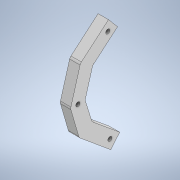
# Autodesk Inventor part: bogie2
Saved by Autodesk Inventor 2020 (Build 240168000, 168)
## iProperties
Created: 2020-05-20
Part Number: bogie2
Material: Generic
Document SubType Name: Modeling
Designer: Manish
Density: 1 g/cm^3
Appearance: Default
Author: Manish
Autodesk Inventor part; units mm, degrees
ref_plane "YZ Plane" through (0, 0, 0) normal (1, 0, 0) x (0, 1, 0)
ref_plane "XZ Plane" through (0, 0, 0) normal (0, 1, 0) x (-1, 0, 0)
ref_plane "XY Plane" through (0, 0, 0) normal (0, 0, 1) x (1, 0, 0)
sketch "Sketch2" plane through (0, 0, 0) normal (1, 0, 0) x (0, 1, 0)
  circle A0 centre (0, 0) radius 3
  line L0 (0, 0) -> (-42.9956, -13.2808)
  line L1 (-42.9956, -13.2808) -> (-74.8971, -51.7814)
  line L2 (0, 0) -> (43.2274, -12.5056)
  line L3 (43.2274, -12.5056) -> (75.6325, -50.5833)
  line L4 (0, 0) -> (-2.961, 9.5861)
  line L5 (0, 0) -> (2.9513, -9.5546)
  line L6 (-42.9956, -13.2808) -> (-46.1884, -2.9442)
  line L7 (-42.9956, -13.2808) -> (-40.0443, -22.8354)
  line L8 (-1.7282, 9.9435) -> (-40.7027, -1.3541)
  line L9 (-30.0445, -19.7466) -> (-1.6206, -10.9668)
  line L10 (-42.9956, -13.2808) -> (-32.8938, -21.6512)
  line L11 (-42.9956, -13.2808) -> (-50.6957, -6.9005)
  line L12 (-32.8938, -21.6512) -> (-64.7954, -60.1517)
  line L13 (-64.7954, -60.1517) -> (-80.1956, -47.3911)
  line L14 (-80.1956, -47.3911) -> (-43.6523, -3.2887)
  line L15 (0, 0) -> (2.779, 9.6061)
  line L16 (0, 0) -> (-2.779, -9.6061)
  line L17 (43.2274, -12.5056) -> (46.0064, -2.8996)
  line L18 (46.0064, -2.8996) -> (40.4484, -22.1117)
  line L19 (1.8176, -10.9359) -> (35.8276, -20.7749)
  line L20 (47.1616, -3.2338) -> (1.6097, 9.9444)
  line L21 (43.2274, -12.5056) -> (50.8429, -6.0246)
  line L22 (43.2274, -12.5056) -> (35.6119, -18.9867)
  line L23 (75.6325, -50.5833) -> (83.2481, -44.1023)
  line L24 (83.2481, -44.1023) -> (68.017, -57.0643)
  line L25 (68.017, -57.0643) -> (38.7295, -22.65)
  line L26 (83.2481, -44.1023) -> (50.0635, -5.1088)
  arc A1 (-40.7027, -1.3541) -> (-43.6523, -3.2887) centre (-39.0322, -7.1169) ccw
  arc A2 (-30.0445, -19.7466) -> (-32.8938, -21.6512) centre (-28.2737, -25.4793) ccw
  arc A3 (1.6097, 9.9444) -> (-1.7282, 9.9435) centre (-0.0577, 4.1807) ccw
  arc A4 (1.8176, -10.9359) -> (-1.6206, -10.9668) centre (0.1501, -16.6995) ccw
  arc A5 (50.0635, -5.1088) -> (47.1616, -3.2338) centre (45.4942, -8.9974) ccw
  arc A6 (38.7295, -22.65) -> (35.8276, -20.7749) centre (34.1601, -26.5386) ccw
  point P0 (2.6602, -14.5039)
  point P1 (16.281, 0.1411)
  point P2 (-48.294, -8.8905)
  dimension "d37" = 6
  dimension "d38" = 45
  dimension "d39" = 10
  dimension "d40" = 20
  dimension "d41" = 50
  dimension "d42" = 10
  dimension "d43" = 10
  dimension "d44" = 10
  dimension "d45" = 20
  dimension "d46" = 10
  dimension "d47" = 10
  dimension "d48" = 10
  dimension "d49" = 20
  dimension "d50" = 6
  dimension "d51" = 6
  dimension "d52" = 50
  dimension "d53" = 10
  dimension "d54" = 1
  dimension "d55" = 33.466
  dimension "d56" = 66.767
  dimension "d57" = 99.956
  dimension "d58" = 75.5671
  dimension "d59" = 77.0952
  dimension "d60" = 22.3248
  dimension "d61" = 74.7699
  dimension "d62" = 42.1891
  constraints: 54 end point, 15 point on line, 14 perpendicular, 12 point on circle, 12 tangent, 7 centre point, 4 equal radius, 3 equal length, 1 coincident
  measures "d37" diameter of A0
  measures "d38" distance between parallel lines of L5 L7
  measures "d39" distance of L0.end L11.end
  measures "d40" distance of L13.start L13.end
  measures "d41" distance between parallel lines of L11 L13
  measures "d42" distance of L16.start L15.end
  measures "d43" distance of L16.start L16.end
  measures "d44" distance of L17.start L17.end
  measures "d45" distance of L17.end L18.end
  measures "d46" distance of L17.start L21.end
  measures "d47" distance of L17.start L22.end
  measures "d48" distance of L3.end L24.start
  measures "d49" distance of L24.start L25.start
  measures "d50" radius of A1
  measures "d51" radius of A3
  measures "d52" distance between parallel lines of L24 L22
  measures "d53" distance between parallel lines of L9 L0
  measures "d54" angle of L0 L8
  measures "d55" angle of L17 L24
  measures "d56" angle of L5 L23
  measures "d57" angle of L10 L23
  measures "d58" distance from line of L24.start L8
  measures "d59" distance from line of point (16.281, 0.141) L24
  measures "d60" distance from line of point (16.281, 0.141) L26
  measures "d61" distance from line of point (2.66, -14.504) L24
  measures "d62" distance from line of point (2.66, -14.504) L26
extrude "Extrusion1" add sketch "Sketch2" along normal blind 15
sketch "Sketch3" plane through (15, 0, 0) normal (1, 0, 0) x (0, 0, -1)
  circle A0 centre (0, 0) radius 3
  line L0 (47.3911, -80.1956) -> (60.1517, -64.7954) projected
  line L1 (3.2887, -43.6523) -> (47.3911, -80.1956) projected
  circle A1 centre (46.0713, -66.1152) radius 3
  line L2 (57.0643, 68.017) -> (44.1023, 83.2481) projected
  line L3 (44.1023, 83.2481) -> (5.1088, 50.0635) projected
  circle A2 centre (42.9678, 69.1515) radius 3
  dimension "d65" = 6
  dimension "d66" = 10
  dimension "d67" = 10
  dimension "d68" = 6
  dimension "d69" = 10
  dimension "d70" = 10
  dimension "d71" = 6
  constraints: 3 centre point, 3 coincident
  measures "d65" diameter of A0
  measures "d66" distance from line of point (46.071, -66.115) L0
  measures "d67" distance from line of L1 point (46.071, -66.115)
  measures "d68" diameter of A1
  measures "d69" distance from line of point (42.968, 69.152) L2
  measures "d70" distance from line of point (42.968, 69.152) L3
  measures "d71" diameter of A2
extrude "Extrusion2" cut sketch "Sketch3" against normal through all
body "Solid1"
